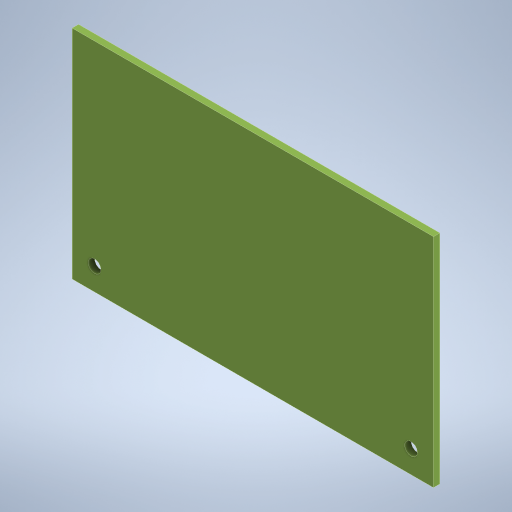
# Autodesk Inventor part: devre kartı
Saved by Autodesk Inventor 2023.2 (Build 272271000, 271)
## iProperties
Created: 2022-12-11
Part Number: devre kartı
Material: Generic
Document SubType Name: Modeling
Designer: omrfrkmll
Density: 1 g/cm^3
Appearance: Olive Green
Author: omrfrkmll
Autodesk Inventor part; units mm, degrees
ref_plane "YZ Plane" through (0, 0, 0) normal (1, 0, 0) x (0, 1, 0)
ref_plane "XZ Plane" through (0, 0, 0) normal (0, 1, 0) x (-1, 0, 0)
ref_plane "XY Plane" through (0, 0, 0) normal (0, 0, 1) x (1, 0, 0)
sketch "Sketch1" plane through (0, 0, 0) normal (0, 0, 1) x (1, 0, 0)
  line L0 (0, 10.3253) -> (0, -8.0216)
  line L1 (-8.0216, 0) -> (9.2969, 0)
  line L2 (-28.25, 17) -> (28.25, 17)
  line L3 (28.25, 17) -> (28.25, -17)
  line L4 (28.25, -17) -> (-28.25, -17)
  line L5 (-28.25, -17) -> (-28.25, 17)
  circle A0 centre (-24.75, -13.5) radius 1
  circle A1 centre (24.75, -13.5) radius 1
  point P0 (0, 0)
  dimension "d0" = 56.5
  dimension "d1" = 34
  dimension "d6" = 3.5
  dimension "d7" = 2
  dimension "d8" = 49.5
  constraints: 12 end point, 3 horizontal, 2 centre point, 2 parallel, 2 vertical, 1 perpendicular, 1 symmetric about line, 3 other
  measures "d0" distance between parallel lines of L3 L5
  measures "d1" distance between parallel lines of L4 L2
  measures "d6" distance from line of L4 A0.centre
  measures "d7" diameter of A0
  measures "d8" distance of A1.centre A0.centre
extrude "Extrusion1" add sketch "Sketch1" along normal blind 1
body "Solid1"
